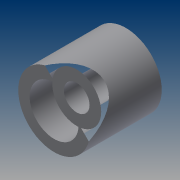
# Autodesk Inventor part: axle
Saved by Autodesk Inventor 2015 SP1 (Build 190203100, 203)
## iProperties
Created: 2015-04-30
Part Number: axle
Material: Generic
Document SubType Name: Modeling
Designer: Trevor
Density: 1 g/cm^3
Appearance: Default
Author: Trevor
Autodesk Inventor part; units mm, degrees
ref_plane "YZ Plane" through (0, 0, 0) normal (1, 0, 0) x (0, 1, 0)
ref_plane "XZ Plane" through (0, 0, 0) normal (0, 1, 0) x (-1, 0, 0)
ref_plane "XY Plane" through (0, 0, 0) normal (0, 0, 1) x (1, 0, 0)
sketch "Sketch1" plane through (0, 0, 0) normal (0, 0, 1) x (1, 0, 0)
  circle A0 centre (0, 0) radius 4.7625
  line L0 (-3.3676, -3.3676) -> (3.3676, -3.3676)
  line L1 (3.3676, -3.3676) -> (3.3676, 3.3676)
  line L2 (3.3676, 3.3676) -> (-3.3676, 3.3676)
  line L3 (-3.3676, 3.3676) -> (-3.3676, -3.3676)
  line L4 (-3.3676, -3.3676) -> (3.3676, 3.3676) construction
  line L5 (3.3676, -3.3676) -> (-3.3676, 3.3676) construction
  dimension "d3" = 6.7352
  constraints: 12 end point, 2 midpoint, 2 parallel, 2 perpendicular, 1 coincident, 1 horizontal, 3 other
  measures "d3" distance of L1.end L2.end
extrude "Extrusion1" add sketch "Sketch1" along normal blind 9.525
hole "Hole1" at (0, 0, 9.525) direction (0, 0, -1) diameter 3.4036 end through all counterbore diameter 6.5024 counterbore depth 2.9972 clearance for "Socket Head Cap Screw" size "M3" standard "Ansi Metric M Profile"
equation "\"d3\" = l_key"
equation "\"d1\" = 2 * t"
equation "\"l_key\" = 6.735192"
equation "\"t\" = 4.7625"
body "Solid1"
